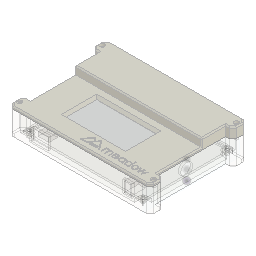
GNSS_Tracker_Enclosure (Autodesk Fusion 360 design; units mm, degrees)
Autodesk Fusion 360 part; units mm, degrees
note: some values were not read from the file. Set by a fixed rule: which sketch regions a step uses.
(part 1 of 2)
sketch "Sketch1" plane through (0, 0, 0) normal (0, 0, 1) x (1, 0, 0) in component "GNSS_PCB"
  line L0 (50, 37.5) -> (-50, 37.5)
  line L1 (-50, 37.5) -> (-50, -37.5)
  line L2 (-50, -37.5) -> (50, -37.5)
  line L3 (50, -37.5) -> (50, 37.5)
  line L4 (50, 37.5) -> (-50, -37.5) construction
  line L5 (-50, 37.5) -> (50, -37.5) construction
  line L6 (0, 37.5) -> (0, -37.5) construction
  line L7 (-50, 0) -> (50, 0) construction
  line L8 (-30.5, 8.425) -> (30.5, 8.425)
  line L9 (30.5, 8.425) -> (30.5, -31.075)
  line L10 (30.5, -31.075) -> (-30.5, -31.075)
  line L11 (-30.5, -31.075) -> (-30.5, 8.425)
  line L12 (-27.5, 1.425) -> (22, 1.425)
  line L13 (22, 1.425) -> (22, -24.075)
  line L14 (22, -24.075) -> (-27.5, -24.075)
  line L15 (-27.5, -24.075) -> (-27.5, 1.425)
  line L16 (-38.5, 35.825) -> (38.5, 35.825)
  line L17 (38.5, 35.825) -> (38.5, 15.175)
  line L18 (38.5, 15.175) -> (-38.5, 15.175)
  line L19 (-38.5, 15.175) -> (-38.5, 35.825)
  line L20 (-33, -37.5) -> (-33, 37.5) construction
  line L21 (40, -37.5) -> (40, 37.5) construction
  line L22 (-28.5, -30.1) -> (-37.5, -30.1)
  line L23 (-37.5, -30.1) -> (-37.5, -37.5)
  line L24 (-37.5, -37.5) -> (-28.5, -37.5)
  line L25 (-28.5, -37.5) -> (-28.5, -30.1)
  line L26 (-28.5, -30.1) -> (-37.5, -37.5) construction
  line L27 (-37.5, -30.1) -> (-28.5, -37.5) construction
  line L28 (42.75, -28.5) -> (37.25, -28.5)
  line L29 (37.25, -28.5) -> (37.25, -40.5)
  line L30 (37.25, -40.5) -> (42.75, -40.5)
  line L31 (42.75, -40.5) -> (42.75, -28.5)
  line L32 (42.75, -28.5) -> (37.25, -40.5) construction
  line L33 (37.25, -28.5) -> (42.75, -40.5) construction
  line L34 (50, -4) -> (-50, -4) construction
  line L35 (-30.5, 3.275) -> (30.5, 3.275)
  line L36 (30.5, 3.275) -> (30.5, -25.925)
  line L37 (30.5, -25.925) -> (-30.5, -25.925)
  line L38 (-30.5, -25.925) -> (-30.5, 3.275)
  point P0 (-47.5, 35)
  point P1 (47.5, 35)
  point P2 (47.5, -35)
  point P3 (-47.5, -35)
  point P4 (-33, -33.8)
  point P5 (40, -34.5)
  dimension "d6" = 75
  dimension "d8" = 100
  dimension "d9" = 2.5
  dimension "d10" = 2.5
  dimension "d19" = 61
  dimension "d20" = 39.5
  dimension "d21" = 30.5
  dimension "d22" = 8.425
  dimension "d23" = 49.5
  dimension "d24" = 25.5
  dimension "d25" = 7
  dimension "d26" = 3
  dimension "d30" = 77
  dimension "d31" = 20.65
  dimension "d32" = 38.5
  dimension "d35" = 35.825
  dimension "d38" = 17
  dimension "d39" = 10
  dimension "d43" = 9
  dimension "d44" = 7.4
  dimension "d45" = 7.4
  dimension "d49" = 5.5
  dimension "d50" = 12
  dimension "d51" = 9
  dimension "d74" = 61
  dimension "d75" = 29.2
  dimension "d76" = 5.15
  constraint horizontal L0
  constraint perpendicular L0 L1
  constraint parallel L0 L2
  constraint parallel L1 L3
  constraint coincident L4 origin
  constraint coincident L5 origin
  constraint midpoint L0 L6.start
  constraint midpoint L2 L6.end
  constraint midpoint L1 L7.start
  constraint midpoint L3 L7.end
  constraint symmetric P0 P1 L6
  constraint symmetric P1 P2 L7
  constraint symmetric P0 P3 L7
  constraint horizontal L8
  constraint vertical L9
  constraint horizontal L10
  constraint vertical L11
  constraint horizontal L12
  constraint vertical L13
  constraint horizontal L14
  constraint vertical L15
  constraint horizontal L16
  constraint vertical L17
  constraint horizontal L18
  constraint vertical L19
  constraint coincident L2 L20.start
  constraint coincident L0 L20.end
  constraint perpendicular L0 L20
  constraint coincident L2 L21.start
  constraint coincident L0 L21.end
  constraint perpendicular L0 L21
  constraint horizontal L22
  constraint perpendicular L22 L23
  constraint parallel L22 L24
  constraint parallel L23 L25
  constraint coincident L26 P4
  constraint coincident L27 P4
  constraint coincident L20 P4
  constraint horizontal L28
  constraint perpendicular L28 L29
  constraint parallel L28 L30
  constraint parallel L29 L31
  constraint coincident L32 P5
  constraint coincident L33 P5
  constraint coincident L21 P5
  constraint coincident L3 L34.start
  constraint coincident L1 L34.end
  constraint perpendicular L1 L34
  constraint horizontal L35
  constraint vertical L36
  constraint horizontal L37
  constraint vertical L38
  constraint coincident L11 L35.start
  measures "d6" distance of L0.end L1.end
  measures "d8" distance of L0.start L0.end
  measures "d9" distance of L0 P0
  measures "d10" distance of L1 P0
  measures "d19" distance of L8.start L8.end
  measures "d20" distance of L8.start L10.end
  measures "d21" distance of L6 L11
  measures "d22" distance of L7 L8
  measures "d23" distance of L12.start L12.end
  measures "d24" distance of L12.start L14.end
  measures "d25" distance of L8 L12
  measures "d26" distance of L11 L15
  measures "d30" distance of L16.start L16.end
  measures "d31" distance of L16.start L18.end
  measures "d32" distance of L6 L19
  measures "d35" distance of L7 L16
  measures "d38" distance of L1 L20
  measures "d39" distance of L3 L21
  measures "d43" distance of L23.end L24.end
  measures "d44" distance of L22.end L23.end
  measures "d45" distance of L2 L22
  measures "d49" distance of L29.end L30.end
  measures "d50" distance of L28.end L29.end
  measures "d51" distance of L2 L28
  measures "d74" distance of L35.start L35.end
  measures "d75" distance of L35.start L37.end
  measures "d76" distance of L8 L35
extrude "Extrude1" add sketch "Sketch1" along normal blind 1.7 contours L0 L1 L2 L3 L8 L9 L10 L11 L22 L23 L25 L28 L29 L31 L36 L38 | L2 L28 L29 L31 | L2 L10 L11 L22 L23 L24 L25 | L9 L10 L11 L22 L25 L37 | L10 L11 L22 L25 | L9 L11 L35 L36 L37 L38 | L8 L9 L11 L35 | L12 L13 L14 L15 | L16 L17 L18 L19 makes body 1 in component "GNSS_PCB"
sketch "Sketch2" plane through (0, 0, 1.7) normal (0, 0, 1) x (-1, 0, 0) in component "GNSS_PCB"
  line L0 (50, 37.5) -> (-50, 37.5)
  line L1 (-50, 37.5) -> (-50, -37.5)
  line L2 (-50, -37.5) -> (50, -37.5)
  line L3 (50, -37.5) -> (50, 37.5)
  line L4 (-37.25, 40.5) -> (-42.75, 40.5)
  line L5 (-37.25, 28.5) -> (-37.25, 40.5)
  line L6 (-42.75, 40.5) -> (-42.75, 28.5)
  line L7 (-40, 37.5) -> (-40, -37.5)
  line L8 (-38.5, -15.175) -> (38.5, -15.175)
  line L9 (-38.5, -35.825) -> (-38.5, -15.175)
  line L10 (38.5, -15.175) -> (38.5, -35.825)
  line L11 (38.5, -35.825) -> (-38.5, -35.825)
  line L12 (-42.75, 28.5) -> (-37.25, 28.5)
  point P0 (47.5, 35)
  point P1 (47.5, -35)
  point P2 (-47.5, -35)
  point P3 (-47.5, 35)
extrude "Extrude2" add sketch "Sketch2" along normal blind 18.5 contours L8 L9 L10 L11 bodies 1 in component "GNSS_PCB"
extrude "Extrude3" add sketch "Sketch2" along normal blind 8.5 contours L0 L5 L7 L12 | L0 L4 L5 L6 | L0 L6 L7 L12 bodies 1 in component "GNSS_PCB"
fillet "Fillet1" radius 10.325 1 edges at (0, 15.175, 20.2) on bodies 1 in component "GNSS_PCB"
fillet "Fillet2" radius 10.325 1 edges at (0, 35.825, 20.2) on bodies 1 in component "GNSS_PCB"
ref_plane "WorkPlane1" through (-5, 0, 3.6) normal (0, 0, 1) x (-1, 0, 0) in component "GNSS_PCB"
sketch "Sketch3" plane through (0, 0, 3.6) normal (0, 0, 1) x (1, 0, 0) in component "GNSS_PCB"
  line L0 (-28.5, -30.1) -> (-37.5, -30.1)
  line L1 (-37.5, -30.1) -> (-37.5, -37.5)
  line L2 (-28.5, -37.5) -> (-28.5, -30.1)
  line L3 (-50, -37.5) -> (50, -37.5)
extrude "Extrude4" add sketch "Sketch3" along normal blind 3.4 separate body makes body 2 in component "GNSS_PCB"
ref_plane "WorkPlane2" through (0, 0, 12.7) normal (0, 0, 1) x (-1, 0, 0) in component "GNSS_PCB"
sketch "Sketch4" plane through (0, 0, 12.7) normal (0, 0, 1) x (1, 0, 0) in component "GNSS_PCB"
  line L0 (-30.5, 8.425) -> (30.5, 8.425)
  line L1 (-30.5, -31.075) -> (-30.5, 8.425)
  line L2 (30.5, 8.425) -> (30.5, -31.075)
  line L3 (30.5, -31.075) -> (-30.5, -31.075)
extrude "Extrude5" add sketch "Sketch4" along normal blind 1.7 separate body makes body 3 in component "GNSS_PCB"
sketch "Sketch5" plane through (0, 0, 14.4) normal (0, 0, 1) x (-1, 0, 0) in component "GNSS_PCB"
  line L0 (-30.5, 31.075) -> (-30.5, -8.425)
  line L1 (-30.5, -8.425) -> (30.5, -8.425)
  line L2 (30.5, -8.425) -> (30.5, 31.075)
  line L3 (30.5, 31.075) -> (-30.5, 31.075)
sketch "Sketch6" plane through (0, 0, 14.4) normal (0, 0, 1) x (-1, 0, 0) in component "GNSS_PCB"
  line L0 (30.5, -3.275) -> (-30.5, -3.275)
  line L1 (-30.5, 25.925) -> (30.5, 25.925)
  line L2 (30.5, 25.925) -> (30.5, -3.275)
  line L3 (-30.5, -3.275) -> (-30.5, 25.925)
extrude "Extrude6" add sketch "Sketch6" along normal blind 1.3 separate body makes body 4 in component "GNSS_PCB"
sketch "Sketch7" plane through (0, 0, 15.7) normal (0, 0, 1) x (-1, 0, 0) in component "GNSS_PCB"
  line L0 (-30.5, -3.275) -> (30.5, -3.275)
  line L1 (30.5, -3.275) -> (30.5, 25.925)
  line L2 (30.5, 25.925) -> (-30.5, 25.925)
  line L3 (-30.5, 25.925) -> (-30.5, -3.275)
  line L4 (-22, 24.075) -> (27.5, 24.075)
  line L5 (-22, -1.425) -> (-22, 24.075)
  line L6 (27.5, 24.075) -> (27.5, -1.425)
  line L7 (27.5, -1.425) -> (-22, -1.425)
hole "Hole1" at (-47.5, -35, 1.7) at (47.5, -35, 1.7) at (-47.5, 35, 1.7) at (47.5, 35, 1.7) direction (0, 0, -1) diameter 2.1 end through all bodies 1 in component "GNSS_PCB"
ref_plane "WorkPlane1" through (0, 0, -3) normal (0, 0, 1) x (1, 0, 0) in component "GNSS_Enclosure_Bottom"
sketch "Sketch1 (2)" plane through (0, 0, -3) normal (0, 0, 1) x (1, 0, 0) in component "GNSS_Enclosure_Bottom"
  line L0 (-50, -37.5) -> (50, -37.5)
  line L1 (50, -37.5) -> (50, 37.5)
  line L2 (50, 37.5) -> (-50, 37.5)
  line L3 (-50, 37.5) -> (-50, -37.5)
  line L4 (51, -38.5) -> (51, 38.5)
  line L5 (51, 38.5) -> (-51, 38.5)
  line L6 (-51, 38.5) -> (-51, -38.5)
  line L7 (-51, -38.5) -> (51, -38.5)
  line L8 (-53, -40.5) -> (53, -40.5)
  line L9 (53, -40.5) -> (53, 40.5)
  line L10 (53, 40.5) -> (-53, 40.5)
  line L11 (-53, 40.5) -> (-53, -40.5)
  circle A0 centre (-47.5, 35) radius 3.5
  circle A1 centre (47.5, 35) radius 3.5
  circle A2 centre (47.5, -35) radius 3.5
  circle A3 centre (-47.5, -35) radius 3.5
  line L12 (-44, 35) -> (-44, 38.5)
  line L13 (-47.5, 31.5) -> (-51, 31.5)
  line L14 (44, 35) -> (44, 38.5)
  line L15 (47.5, 31.5) -> (51, 31.5)
  line L16 (47.5, -31.5) -> (51, -31.5)
  line L17 (44, -35) -> (44, -38.5)
  line L18 (-47.5, -31.5) -> (-51, -31.5)
  line L19 (-44, -35) -> (-44, -38.5)
  point P0 (47.5, 35)
  point P1 (-47.5, 35)
  point P2 (-47.5, -35)
  point P3 (47.5, -35)
  dimension "d87" = 1
  dimension "d88" = 3
  constraint coincident P1 A0.centre
  constraint tangent L5 A0
  constraint coincident P0 A1.centre
  constraint tangent L5 A1
  constraint coincident P3 A2.centre
  constraint tangent L4 A2
  constraint coincident P2 A3.centre
  constraint tangent L7 A3
  constraint coincident A0 L12.start
  constraint coincident L5 L12.end
  constraint tangent A0 L12
  constraint perpendicular L5 L12
  constraint coincident A0 L13.start
  constraint coincident L6 L13.end
  constraint tangent A0 L13
  constraint perpendicular L6 L13
  constraint coincident A1 L14.start
  constraint coincident L5 L14.end
  constraint tangent A1 L14
  constraint perpendicular L5 L14
  constraint coincident A1 L15.start
  constraint coincident L4 L15.end
  constraint tangent A1 L15
  constraint perpendicular L4 L15
  constraint coincident A2 L16.start
  constraint coincident L4 L16.end
  constraint tangent A2 L16
  constraint perpendicular L4 L16
  constraint coincident A2 L17.start
  constraint coincident L7 L17.end
  constraint tangent A2 L17
  constraint perpendicular L7 L17
  constraint coincident A3 L18.start
  constraint coincident L6 L18.end
  constraint tangent A3 L18
  constraint perpendicular L6 L18
  constraint coincident A3 L19.start
  constraint coincident L7 L19.end
  constraint tangent A3 L19
  constraint perpendicular L7 L19
extrude "Extrude1'" add sketch "Sketch1 (2)" against normal blind 2 separate body contours L0 L3 A3 | L0 L3 L6 L7 A3 | L0 L3 A3 | L0 A3 | L3 A3 | L0 A3 L19 | L0 L7 A3 L19 | L3 L6 A3 L18 | L3 A3 L18 | L0 L1 L2 L3 A0 A1 A2 A3 L12 L13 L14 L15 L16 L17 L18 L19 | L0 L7 L17 L19 | L3 L6 L13 L18 | L0 A2 L17 | L0 L7 A2 L17 | L3 L6 A0 L13 | L3 A0 L13 | L0 L1 A2 | L0 A2 | L0 L1 L4 L7 A2 | L3 A0 | L2 L3 A0 | L2 L3 L5 L6 A0 | L0 L1 A2 | L1 A2 L16 | L2 L3 A0 | L2 A0 L12 | L1 A2 | L1 L4 A2 L16 | L1 L4 L15 L16 | L2 A0 | L2 L5 A0 L12 | L2 L5 L12 L14 | L1 A1 L15 | L1 L4 A1 L15 | L2 L5 A1 L14 | L2 A1 L14 | L1 L2 A1 | L1 A1 | L2 A1 | L1 L2 A1 | L1 L2 L4 L5 A1 | L8 L9 L10 L11 makes body 5 in component "GNSS_Enclosure_Bottom"
extrude "Extrude2'" add sketch "Sketch1 (2)" along normal up to surface (18.7 mm away) bodies 5 in component "GNSS_Enclosure_Bottom"
extrude "Extrude3'" add sketch "Sketch1 (2)" along normal blind 3 contours L0 L3 A3 | L0 L3 L6 L7 A3 | L0 L3 A3 | L0 A3 | L3 A3 | L0 A3 L19 | L0 L7 A3 L19 | L3 L6 A3 L18 | L3 A3 L18 | L0 A2 L17 | L0 L7 A2 L17 | L3 L6 A0 L13 | L3 A0 L13 | L0 L1 A2 | L0 A2 | L0 L1 L4 L7 A2 | L3 A0 | L2 L3 A0 | L2 L3 L5 L6 A0 | L1 A2 L16 | L2 A0 L12 | L1 A2 | L1 L4 A2 L16 | L2 A0 | L2 L5 A0 L12 | L1 A1 L15 | L1 L4 A1 L15 | L2 L5 A1 L14 | L2 A1 L14 | L1 L2 A1 | L1 A1 | L2 A1 | L1 L2 L4 L5 A1 picked at (48.0119, -34.834) picked at (-48.3502, 35.8333) picked at (47.0153, 35.6054) bodies 5 in component "GNSS_Enclosure_Bottom"
sketch "Sketch2 (2)" plane through (0, 0, 0) normal (0, 0, 1) x (-1, 0, 0) in component "GNSS_Enclosure_Bottom"
  line L0 (-50, -37.5) -> (-50, -37.4495)
  arc A0 (-50, -37.4495) -> (-49.9495, -37.5) centre (-47.5, -35) ccw
  line L1 (-49.9495, -37.5) -> (-50, -37.5)
  arc A1 (-44, -35) -> (-47.5, -31.5) centre (-47.5, -35) ccw
  line L2 (-47.5, -31.5) -> (-51, -31.5)
  line L3 (-51, -31.5) -> (-51, -38.5)
  line L4 (-51, -38.5) -> (-44, -38.5)
  line L5 (-44, -38.5) -> (-44, -35)
  point P0 (-47.5, 35)
  point P1 (47.5, 35)
  point P2 (47.5, -35)
  point P3 (-47.5, -35)
hole "Hole1'" at (47.5, -35, 0) at (-47.5, -35, 0) at (47.5, 35, 0) at (-47.5, 35, 0) direction (0, 0, -1) diameter 3 depth 3 tip angle 180 bodies 5 in component "GNSS_Enclosure_Bottom"
sketch "Sketch3 (2)" plane through (0, -40.5, 0) normal (0, -1, 0) x (1, 0, 0) in component "GNSS_Enclosure_Bottom"
  line L0 (-53, 15.7) -> (-53, -5)
  line L1 (-53, -5) -> (53, -5)
  line L2 (53, -5) -> (53, 15.7)
  line L3 (53, 15.7) -> (-53, 15.7)
  line L4 (-37.5, 3.6) -> (-28.5, 3.6)
  line L5 (-28.5, 3.6) -> (-28.5, 7)
  line L6 (-28.5, 7) -> (-37.5, 7)
  line L7 (-37.5, 7) -> (-37.5, 3.6)
  line L8 (37.25, 1.7) -> (42.75, 1.7)
  line L9 (42.75, 1.7) -> (42.75, 10.2)
  line L10 (42.75, 10.2) -> (37.25, 10.2)
  line L11 (37.25, 10.2) -> (37.25, 1.7)
  line L12 (36.25, 11.2) -> (36.25, 0.7)
  line L13 (36.25, 0.7) -> (43.75, 0.7)
  line L14 (43.75, 0.7) -> (43.75, 11.2)
  line L15 (43.75, 11.2) -> (36.25, 11.2)
  line L16 (-33, 7) -> (-33, 3.6) construction
  line L17 (-37.5, 5.3) -> (-28.5, 5.3) construction
  line L18 (-26, 10.3) -> (-40, 10.3)
  line L19 (-40, 10.3) -> (-40, 0.3)
  line L20 (-40, 0.3) -> (-26, 0.3)
  line L21 (-26, 0.3) -> (-26, 10.3)
  line L22 (-26, 10.3) -> (-40, 0.3) construction
  line L23 (-40, 10.3) -> (-26, 0.3) construction
  point P0 (-33, 5.3)
  dimension "d102" = 1
  dimension "d107" = 14
  dimension "d108" = 10
  constraint midpoint L6 L16.start
  constraint midpoint L4 L16.end
  constraint midpoint L7 L17.start
  constraint midpoint L5 L17.end
  constraint horizontal L18
  constraint perpendicular L18 L19
  constraint parallel L18 L20
  constraint parallel L19 L21
  constraint coincident L22 P0
  constraint coincident L23 P0
  constraint midpoint L17 P0
  measures "d107" distance of L19.end L20.end
  measures "d108" distance of L18.end L19.end
extrude "Extrude4'" cut sketch "Sketch3 (2)" against normal up to surface (2 mm away) contours L8 L9 L10 L11 | L12 L13 L14 L15 bodies 5 in component "GNSS_Enclosure_Bottom"
extrude "Extrude5'" cut sketch "Sketch3 (2)" against normal up to surface (2 mm away) contours L4 L5 L6 L7 | L18 L19 L20 L21 bodies 5 in component "GNSS_Enclosure_Bottom"
sketch "Sketch1 (3)" plane through (0, 0, 15.7) normal (0, 0, 1) x (-1, 0, 0) in component "GNSS_Enclosure_Top"
  line L0 (-51, -38.5) -> (-51, 38.5)
  line L1 (-51, 38.5) -> (51, 38.5)
  line L2 (51, 38.5) -> (51, -38.5)
  line L3 (51, -38.5) -> (-51, -38.5)
  line L4 (-53, -40.5) -> (53, -40.5)
  line L5 (53, -40.5) -> (53, 40.5)
  line L6 (53, 40.5) -> (-53, 40.5)
  line L7 (-53, 40.5) -> (-53, -40.5)
  line L8 (-38.5, -35.825) -> (-38.5, -15.175)
  line L9 (38.5, -35.825) -> (-38.5, -35.825)
  line L10 (-38.5, -15.175) -> (38.5, -15.175)
  line L11 (38.5, -15.175) -> (38.5, -35.825)
  line L12 (53, -40.5) -> (-53, -40.5)
  line L13 (53, 40.5) -> (53, -40.5)
  line L14 (-53, -40.5) -> (-53, 40.5)
  line L15 (-53, 40.5) -> (53, 40.5)
  line L16 (53, -10.5) -> (-53, -10.5)
  line L17 (-51, 38.5) -> (-51, -38.5)
  line L18 (-51, -38.5) -> (51, -38.5)
  line L19 (51, -38.5) -> (51, 38.5)
  dimension "d111" = 4.675
  dimension "d112" = 4.675
  constraint coincident L13 L16.start
  constraint coincident L14 L16.end
  constraint perpendicular L14 L16
  measures "d111" distance of L4 L9
  measures "d112" distance of L10 L16
extrude "Extrude1''" add sketch "Sketch1 (3)" along normal blind 2 separate body contours L0 L2 L3 L4 L5 L7 L12 L13 L14 L16 L17 L18 L19 | L0 L1 L2 L5 L6 L7 L13 L14 L15 L16 L17 L19 | L0 L1 L2 L16 L17 L19 makes body 6 in component "GNSS_Enclosure_Top"
sketch "Sketch2 (3)" plane through (0, 0, 17.7) normal (0, 0, 1) x (-1, 0, 0) in component "GNSS_Enclosure_Top"
  line L0 (51, -10.5) -> (51, -38.5)
  line L1 (51, -38.5) -> (-51, -38.5)
  line L2 (-51, -38.5) -> (-51, -10.5)
  line L3 (-51, -10.5) -> (51, -10.5)
  line L4 (-53, 40.5) -> (-53, -40.5)
  line L5 (-53, -40.5) -> (53, -40.5)
  line L6 (53, -40.5) -> (53, 40.5)
  line L7 (53, 40.5) -> (-53, 40.5)
  line L8 (-53, -8.5) -> (53, -8.5)
  dimension "d115" = 2
  constraint coincident L4 L8.start
  constraint coincident L6 L8.end
  constraint perpendicular L6 L8
  measures "d115" distance of L3 L8
sketch "Sketch3 (3)" plane through (53, 0, 0) normal (1, 0, 0) x (0, 1, 0) in component "GNSS_Enclosure_Top"
  line L0 (-40.5, 15.7) -> (40.5, 15.7)
  line L1 (40.5, 15.7) -> (40.5, 17.7)
  line L2 (40.5, 17.7) -> (-40.5, 17.7)
  line L3 (-40.5, 17.7) -> (-40.5, 15.7)
  arc A0 (35.825, 9.875) -> (15.175, 9.875) centre (25.5, 9.875) ccw
  line L4 (25.5, 20.2) -> (40.5, 20.2) construction
  line L5 (40.5, 20.2) -> (40.5, 17.7) construction
  line L6 (25.5, 22.2) -> (42.5, 22.2) construction
  line L7 (42.5, 22.2) -> (42.5, 17.7) construction
  constraint midpoint A0 L4.start
  constraint tangent A0 L4
  constraint perpendicular L1 L4
  constraint coincident L1.end L2.start
  constraint perpendicular L2 L5
extrude "Extrude2''" add sketch "Sketch2 (3)" along normal up to surface (4.5 mm away) contours L4 L5 L6 L8 bodies 6 in component "GNSS_Enclosure_Top"
sketch "Sketch4 (2)" plane through (0, 0, 22.2) normal (0, 0, 1) x (-1, 0, 0) in component "GNSS_Enclosure_Top"
  line L0 (51, -38.5) -> (-51, -38.5)
  line L1 (-51, -38.5) -> (-51, -10.5)
  line L2 (-51, -10.5) -> (51, -10.5)
  line L3 (51, -10.5) -> (51, -38.5)
  line L4 (-53, -8.5) -> (-53, -40.5)
  line L5 (-53, -40.5) -> (53, -40.5)
  line L6 (53, -40.5) -> (53, -8.5)
  line L7 (53, -8.5) -> (-53, -8.5)
extrude "Extrude3''" add sketch "Sketch4 (2)" along normal blind 2 contours L0 L1 L2 L3 | L4 L5 L6 L7 bodies 6 in component "GNSS_Enclosure_Top"
sketch "Sketch4 (3)" plane through (53, 0, 0) normal (1, 0, 0) x (0, 1, 0) in component "GNSS_Enclosure_Bottom"
  line L0 (-40.5, 15.7) -> (-40.5, -5)
  line L1 (-40.5, -5) -> (40.5, -5)
  line L2 (40.5, -5) -> (40.5, 15.7)
  line L3 (40.5, 15.7) -> (-40.5, 15.7)
  line L4 (-4, 0) -> (-4, 15.7) construction
  point P0 (-4, 0)
  point P1 (-4, 8.2)
  dimension "d124" = 8.2
  constraint coincident P0 L4.start
  constraint coincident L3 L4.end
  constraint perpendicular L3 L4
  constraint coincident L4 P1
  measures "d124" distance of P0 P1
hole "Hole2" at (53, -4, 8.2) direction (-1, 0, 0) diameter 10 depth 2 tip angle 180 bodies 5 in component "GNSS_Enclosure_Bottom"
sketch "Sketch5 (2)" plane through (0, 0, -5) normal (0, 0, -1) x (1, 0, 0) in component "GNSS_Enclosure_Bottom"
  line L0 (-53, 40.5) -> (-53, -40.5)
  line L1 (-53, -40.5) -> (53, -40.5)
  line L2 (53, -40.5) -> (53, 40.5)
  line L3 (53, 40.5) -> (-53, 40.5)
  line L4 (-53, 40.5) -> (-53, -40.5)
  line L5 (53, -40.5) -> (53, 40.5)
  line L6 (59, -40.5) -> (59, 40.5) construction
  line L7 (-59, 40.5) -> (-59, -40.5) construction
  line L8 (59, -40.5) -> (53, -40.5) construction
  line L9 (59, 40.5) -> (53, 40.5) construction
  line L10 (-59, -40.5) -> (-53, -40.5) construction
  line L11 (-59, 40.5) -> (-53, 40.5) construction
  line L12 (59, -28.5) -> (53, -28.5) construction
  line L13 (56, -40.5) -> (56, -28.5) construction
  line L14 (53, -40.5) -> (59, -40.5)
  line L15 (59, -28.5) -> (59, -40.5)
  line L16 (59, -28.5) -> (53, -28.5)
  line L17 (59, 28.5) -> (53, 28.5)
  line L18 (59, 28.5) -> (59, 40.5)
  line L19 (59, 40.5) -> (53, 40.5)
  line L20 (-59, -28.5) -> (-53, -28.5)
  line L21 (-59, 28.5) -> (-53, 28.5)
  line L22 (-53, -40.5) -> (-59, -40.5)
  line L23 (-59, -28.5) -> (-59, -40.5)
  line L24 (-59, 28.5) -> (-59, 40.5)
  line L25 (-59, 40.5) -> (-53, 40.5)
  line L26 (56, 28.5) -> (56, 40.5) construction
  line L27 (59, 34.5) -> (53, 34.5) construction
  line L28 (-56, -40.5) -> (-56, -28.5) construction
  line L29 (-56, 28.5) -> (-56, 40.5) construction
  point P0 (56, -34.5)
  point P1 (-56, -34.5)
  point P2 (-56, 34.5)
  point P3 (56, 34.5)
  dimension "d129" = 6
  dimension "d130" = 6
  dimension "d131" = 12
  dimension "d132" = 12
  dimension "d133" = 12
  dimension "d134" = 12
  constraint coincident L1.end L2.start
  constraint perpendicular L5 L8
  constraint coincident L2.end L3.start
  constraint perpendicular L5 L9
  constraint coincident L0.end L1.start
  constraint perpendicular L4 L10
  constraint coincident L0.start L3.end
  constraint perpendicular L4 L11
  constraint coincident L6 L12.start
  constraint coincident L2 L12.end
  constraint perpendicular L2 L12
  constraint midpoint L8 L13.start
  constraint midpoint L12 L13.end
  constraint midpoint L13 P0
  constraint coincident L6 L17.start
  constraint coincident L5 L17.end
  constraint perpendicular L5 L17
  constraint coincident L7 L20.start
  constraint coincident L0 L20.end
  constraint perpendicular L0 L20
  constraint coincident L7 L21.start
  constraint coincident L4 L21.end
  constraint perpendicular L4 L21
  constraint midpoint L17 L26.start
  constraint midpoint L9 L26.end
  constraint midpoint L18 L27.start
  constraint coincident L5 L27.end
  constraint perpendicular L5 L27
  constraint midpoint L10 L28.start
  constraint midpoint L20 L28.end
  constraint midpoint L21 L29.start
  constraint midpoint L25 L29.end
  constraint midpoint L28 P1
  constraint midpoint L29 P2
  constraint midpoint L26 P3
  measures "d131" distance of L8 L12
  measures "d132" distance of L9 L17
  measures "d133" distance of L10 L20
  measures "d134" distance of L11 L21
extrude "Extrude6'" add sketch "Sketch5 (2)" against normal up to surface (20.7 mm away) contours L0 L4 L21 L24 L25 | L2 L5 L17 L18 L19 | L0 L4 L20 L22 L23 | L2 L5 L14 L15 L16 bodies 5 in component "GNSS_Enclosure_Bottom"
chamfer "Chamfer1" distance 3 angle 45 8 edges at (59, -40.5, 5.35) (59, 40.5, 5.35) (59, 28.5, 5.35) (59, -28.5, 5.35) (-59, -40.5, 5.35) (-59, -28.5, 5.35) (-59, 28.5, 5.35) (-59, 40.5, 5.35) on bodies 5 in component "GNSS_Enclosure_Bottom"
sketch "Sketch6 (2)" plane through (0, 0, 15.7) normal (0, 0, 1) x (-1, 0, 0) in component "GNSS_Enclosure_Bottom"
  line L0 (-51, -38.5) -> (-51, 38.5)
  line L1 (-51, 38.5) -> (51, 38.5)
  line L2 (51, 38.5) -> (51, -38.5)
  line L3 (51, -38.5) -> (-51, -38.5)
  line L4 (56, -40.5) -> (59, -37.5)
  line L5 (59, -37.5) -> (59, -31.5)
  line L6 (59, -31.5) -> (56, -28.5)
  line L7 (56, -28.5) -> (53, -28.5)
  line L8 (53, -28.5) -> (53, 28.5)
  line L9 (53, 28.5) -> (56, 28.5)
  line L10 (56, 28.5) -> (59, 31.5)
  line L11 (59, 31.5) -> (59, 37.5)
  line L12 (59, 37.5) -> (56, 40.5)
  line L13 (56, 40.5) -> (-56, 40.5)
  line L14 (-56, 40.5) -> (-59, 37.5)
  line L15 (-59, 37.5) -> (-59, 31.5)
  line L16 (-59, 31.5) -> (-56, 28.5)
  line L17 (-56, 28.5) -> (-53, 28.5)
  line L18 (-53, 28.5) -> (-53, -28.5)
  line L19 (-53, -28.5) -> (-56, -28.5)
  line L20 (-56, -28.5) -> (-59, -31.5)
  line L21 (-59, -31.5) -> (-59, -37.5)
  line L22 (-59, -37.5) -> (-56, -40.5)
  line L23 (-56, -40.5) -> (56, -40.5)
  line L24 (-53, -28.5) -> (-53, -40.5)
  line L25 (53, -28.5) -> (53, -40.5)
  point P0 (-56, 34.5)
  point P1 (-56, -34.5)
  point P2 (56, -34.5)
  point P3 (56, 34.5)
  point P4 (-53, -40.5)
  point P5 (53, -40.5)
  constraint coincident L18.end L19.start
  constraint coincident P4 L24.end
  constraint coincident L7.end L8.start
  constraint coincident P5 L25.end
hole "Hole3" at (-56, -34.5, 15.7) at (-56, 34.5, 15.7) at (56, -34.5, 15.7) at (56, 34.5, 15.7) direction (0, 0, -1) diameter 3 depth 3 tip angle 180 bodies 5 in component "GNSS_Enclosure_Bottom"
chamfer "Chamfer2" distance 0.2 distance2 3 8 edges at (-57.3985, 35.0424, 15.7) (54.6015, 35.0424, 15.7) (-48.8985, 35.5424, 0) (-57.3985, -33.9576, 15.7) (54.6015, -33.9576, 15.7) (46.1015, 35.5424, 0) (46.1015, -34.4576, 0) (-48.8985, -34.4576, 0) measured on face at (54.063, -38.254, 15.7) measured on face at (54.063, -38.254, 15.7) measured on face at (-48.9483, 32.2535, 0) measured on face at (54.063, -38.254, 15.7) measured on face at (54.063, -38.254, 15.7) measured on face at (48.9483, 32.2535, 0) measured on face at (48.9483, -32.2535, 0) measured on face at (-50.3319, -34.9626, 0) on bodies 5 in component "GNSS_Enclosure_Bottom"
sketch "Sketch5 (3)" plane through (0, 0, 15.7) normal (0, 0, -1) x (1, 0, 0) in component "GNSS_Enclosure_Top"
  line L0 (-51, -38.5) -> (-51, -10.5)
  line L1 (-51, -10.5) -> (51, -10.5)
  line L2 (51, -10.5) -> (51, -38.5)
  line L3 (51, -38.5) -> (-51, -38.5)
  line L4 (53, -40.5) -> (53, 40.5)
  line L5 (53, 40.5) -> (-53, 40.5)
  line L6 (-53, 40.5) -> (-53, -40.5)
  line L7 (-53, -40.5) -> (53, -40.5)
  circle A0 centre (-56, 34.5) radius 1.7
  circle A1 centre (-56, -34.5) radius 1.7
  line L8 (51, -38.5) -> (51, 38.5)
  line L9 (51, 38.5) -> (-51, 38.5)
  line L10 (-51, 38.5) -> (-51, -38.5)
  line L11 (-51, -38.5) -> (51, -38.5)
  line L12 (-56, -40.5) -> (-59, -37.5)
  line L13 (-59, -37.5) -> (-59, -31.5)
  line L14 (-59, -31.5) -> (-56, -28.5)
  line L15 (-56, -28.5) -> (-53, -28.5)
  line L16 (-53, -28.5) -> (-53, 28.5)
  line L17 (-53, 28.5) -> (-56, 28.5)
  line L18 (-56, 28.5) -> (-59, 31.5)
  line L19 (-59, 31.5) -> (-59, 37.5)
  line L20 (-59, 37.5) -> (-56, 40.5)
  line L21 (-56, 40.5) -> (56, 40.5)
  line L22 (56, 40.5) -> (59, 37.5)
  line L23 (59, 37.5) -> (59, 31.5)
  line L24 (59, 31.5) -> (56, 28.5)
  line L25 (56, 28.5) -> (53, 28.5)
  line L26 (53, 28.5) -> (53, -28.5)
  line L27 (53, -28.5) -> (56, -28.5)
  line L28 (56, -28.5) -> (59, -31.5)
  line L29 (59, -31.5) -> (59, -37.5)
  line L30 (59, -37.5) -> (56, -40.5)
  line L31 (56, -40.5) -> (-56, -40.5)
  circle A2 centre (56, -34.5) radius 1.7
  circle A3 centre (56, 34.5) radius 1.7
extrude "Extrude4''" add sketch "Sketch5 (3)" against normal up to surface (2 mm away) contours L4 L21 L22 L23 L24 L25 | L6 L17 L18 L19 L20 L21 | A0 | A3 bodies 6 in component "GNSS_Enclosure_Top"
extrude "Extrude5''" add sketch "Sketch6 (2)" along normal up to surface (8.5 mm away) contours L4 L5 L6 L7 L23 L25 | L19 L20 L21 L22 L23 L24 bodies 6 in component "GNSS_Enclosure_Top"
sketch "Sketch6 (3)" plane through (0, 0, 15.7) normal (0, 0, 1) x (1, 0, 0) in component "GNSS_Enclosure_Top"
sketch "Sketch7 (2)" plane through (0, 0, 17.7) normal (0, 0, 1) x (-1, 0, 0) in component "GNSS_Enclosure_Top"
  line L0 (-53, -8.5) -> (53, -8.5)
  line L1 (53, -8.5) -> (53, 28.5)
  line L2 (53, 28.5) -> (56, 28.5)
  line L3 (56, 28.5) -> (59, 31.5)
  line L4 (59, 31.5) -> (59, 37.5)
  line L5 (59, 37.5) -> (56, 40.5)
  line L6 (56, 40.5) -> (-56, 40.5)
  line L7 (-56, 40.5) -> (-59, 37.5)
  line L8 (-59, 37.5) -> (-59, 31.5)
  line L9 (-59, 31.5) -> (-56, 28.5)
  line L10 (-56, 28.5) -> (-53, 28.5)
  line L11 (-53, 28.5) -> (-53, -8.5)
  point P0 (56, 34.5)
  point P1 (-56, 34.5)
sketch "Sketch8" plane through (0, 0, 24.2) normal (0, 0, 1) x (-1, 0, 0) in component "GNSS_Enclosure_Top"
  line L0 (53, -8.5) -> (-53, -8.5)
  line L1 (-53, -8.5) -> (-53, -28.5)
  line L2 (-53, -28.5) -> (-56, -28.5)
  line L3 (-56, -28.5) -> (-59, -31.5)
  line L4 (-59, -31.5) -> (-59, -37.5)
  line L5 (-59, -37.5) -> (-56, -40.5)
  line L6 (-56, -40.5) -> (56, -40.5)
  line L7 (56, -40.5) -> (59, -37.5)
  line L8 (59, -37.5) -> (59, -31.5)
  line L9 (59, -31.5) -> (56, -28.5)
  line L10 (56, -28.5) -> (53, -28.5)
  line L11 (53, -28.5) -> (53, -8.5)
  point P0 (56, -34.5)
  point P1 (-56, -34.5)
hole "Hole1''" at (-56, 34.5, 24.2) at (56, 34.5, 24.2) direction (0, 0, -1) diameter 2.3 depth 8.6 tip angle 180 counterbore diameter 4 counterbore depth 2 bodies 6 in component "GNSS_Enclosure_Top"
hole "Hole2'" at (-56, -34.5, 17.7) at (56, -34.5, 17.7) direction (0, 0, -1) diameter 2.3 depth 2 tip angle 180 counterbore diameter 4 counterbore depth 1 bodies 6 in component "GNSS_Enclosure_Top"
sketch "Sketch9" plane through (0, 0, 17.7) normal (0, 0, 1) x (-1, 0, 0) in component "GNSS_Enclosure_Top"
  circle A0 centre (56, 34.5) radius 2
  circle A1 centre (-56, 34.5) radius 2
  line L0 (-53, -8.5) -> (53, -8.5)
  line L1 (53, -8.5) -> (53, 28.5)
  line L2 (53, 28.5) -> (56, 28.5)
  line L3 (56, 28.5) -> (59, 31.5)
  line L4 (59, 31.5) -> (59, 37.5)
  line L5 (59, 37.5) -> (56, 40.5)
  line L6 (56, 40.5) -> (-56, 40.5)
  line L7 (-56, 40.5) -> (-59, 37.5)
  line L8 (-59, 37.5) -> (-59, 31.5)
  line L9 (-59, 31.5) -> (-56, 28.5)
  line L10 (-56, 28.5) -> (-53, 28.5)
  line L11 (-53, 28.5) -> (-53, -8.5)
  line L12 (27.5, -1.425) -> (-22, -1.425)
  line L13 (27.5, 24.075) -> (27.5, -1.425)
  line L14 (-22, 24.075) -> (27.5, 24.075)
  line L15 (-22, -1.425) -> (-22, 24.075)
extrude "Extrude6''" cut sketch "Sketch9" against normal up to surface (2 mm away) contours L12 L13 L14 L15 bodies 6 in component "GNSS_Enclosure_Top"
chamfer "Chamfer1'" distance 2 angle 45 4 edges at (-2.75, 1.425, 17.7) (22, -11.325, 17.7) (-2.75, -24.075, 17.7) (-27.5, -11.325, 17.7) on bodies 6 in component "GNSS_Enclosure_Top"
chamfer "Chamfer2'" distance 1 angle 45 25 edges at (59, -34.5, 17.7) (57.5, -30, 17.7) (54.5, -28.5, 17.7) (53, -10, 17.7) (57.5, -39, 17.7) (0, -40.5, 17.7) (-57.5, -39, 17.7) (-59, -34.5, 17.7) (-57.5, -30, 17.7) (-54.5, -28.5, 17.7) (-53, -10, 17.7) (-53, 8.5, 20.95) (-53, 18.5, 24.2) (0, 8.5, 24.2) (-54.5, 28.5, 24.2) (-57.5, 30, 24.2) (-59, 34.5, 24.2) (-57.5, 39, 24.2) (0, 40.5, 24.2) (57.5, 39, 24.2) (59, 34.5, 24.2) (57.5, 30, 24.2) (54.5, 28.5, 24.2) (53, 18.5, 24.2) (53, 8.5, 20.95) on bodies 6 in component "GNSS_Enclosure_Top"
chamfer "Chamfer3" distance 1 angle 45 20 edges at (0, -40.5, -5) (-57.5, -39, -5) (-59, -34.5, -5) (-57.5, -30, -5) (-54.5, -28.5, -5) (-53, 0, -5) (57.5, -39, -5) (59, -34.5, -5) (57.5, -30, -5) (54.5, -28.5, -5) (53, 0, -5) (54.5, 28.5, -5) (57.5, 30, -5) (59, 34.5, -5) (57.5, 39, -5) (0, 40.5, -5) (-57.5, 39, -5) (-59, 34.5, -5) (-57.5, 30, -5) (-54.5, 28.5, -5) on bodies 5 in component "GNSS_Enclosure_Bottom"
sketch "Sketch10" plane through (0, 0, 17.7) normal (0, 0, 1) x (-1, 0, 0) in component "GNSS_Enclosure_Top"
  line L0 (-24, -3.425) -> (-24, 26.075)
  line L1 (-24, 26.075) -> (29.5, 26.075)
  line L2 (29.5, 26.075) -> (29.5, -3.425)
  line L3 (29.5, -3.425) -> (-24, -3.425)
  line L4 (52, -8.5) -> (52, 29.5)
  line L5 (52, 29.5) -> (55.5858, 29.5)
  line L6 (55.5858, 29.5) -> (58, 31.9142)
  line L7 (58, 31.9142) -> (58, 34.5)
  circle A0 centre (56, 34.5) radius 2
  line L8 (58, 34.5) -> (58, 37.0858)
  line L9 (58, 37.0858) -> (55.5858, 39.5)
  line L10 (55.5858, 39.5) -> (-55.5858, 39.5)
  line L11 (-55.5858, 39.5) -> (-58, 37.0858)
  line L12 (-58, 37.0858) -> (-58, 34.5)
  circle A1 centre (-56, 34.5) radius 2
  line L13 (-58, 34.5) -> (-58, 31.9142)
  line L14 (-58, 31.9142) -> (-55.5858, 29.5)
  line L15 (-55.5858, 29.5) -> (-52, 29.5)
  line L16 (-52, 29.5) -> (-52, -8.5)
  line L17 (-52, -8.5) -> (52, -8.5)
  line L18 (-20.2661, 33.2143) -> (-20.2661, 35.8128)
  line L19 (-20.2661, 35.8128) -> (-19.6706, 35.8128)
  line L20 (-19.6706, 35.8128) -> (-19.6706, 33.2294)
  spline S0 degree 3 poles (-19.6706, 33.2294) (-19.6706, 32.473) (-19.1109, 31.8735) (-18.3752, 31.8735) knots 0 0 0 0 1 1 1 1
  spline S1 degree 3 poles (-18.3752, 31.8735) (-17.6395, 31.8735) (-17.0687, 32.4724) (-17.0687, 33.2294) knots 0 0 0 0 1 1 1 1
  line L21 (-17.0687, 33.2294) -> (-17.0687, 35.8107)
  line L22 (-17.0687, 35.8107) -> (-16.4822, 35.8107)
  line L23 (-16.4822, 35.8107) -> (-16.4822, 33.2294)
  spline S2 degree 3 poles (-16.4822, 33.2294) (-16.4822, 32.473) (-15.9046, 31.8735) (-15.1758, 31.8735) knots 0 0 0 0 1 1 1 1
  spline S3 degree 3 poles (-15.1758, 31.8735) (-14.4469, 31.8735) (-13.8755, 32.473) (-13.8755, 33.2294) knots 0 0 0 0 1 1 1 1
  line L24 (-13.8755, 33.2294) -> (-13.8755, 35.8107)
  line L25 (-13.8755, 35.8107) -> (-13.2979, 35.8107)
  line L26 (-13.2979, 35.8107) -> (-13.2979, 31.4079)
  line L27 (-13.2979, 31.4079) -> (-13.8755, 31.4079)
  line L28 (-13.8755, 31.4079) -> (-13.8755, 32.0605)
  spline S4 degree 3 poles (-13.8755, 32.0605) (-14.2016, 31.6114) (-14.7212, 31.3436) (-15.2762, 31.3385) knots 0 0 0 0 1 1 1 1
  spline S5 degree 3 poles (-15.2762, 31.3385) (-15.9326, 31.3381) (-16.5356, 31.7006) (-16.8432, 32.2805) knots 0 0 0 0 1 1 1 1
  spline S6 degree 3 poles (-16.8432, 32.2805) (-17.1409, 31.7167) (-17.7371, 31.3385) (-18.4715, 31.3385) knots 0 0 0 0 1 1 1 1
  spline S7 degree 3 poles (-18.4715, 31.3385) (-19.4953, 31.3378) (-20.2661, 32.1657) (-20.2661, 33.2143) knots 0 0 0 0 1 1 1 1
  line L29 (-25.0333, 34.1831) -> (-25.5229, 34.3592)
  spline S8 degree 3 poles (-25.5229, 34.3592) (-25.2953, 34.978) (-24.5341, 35.8478) (-23.3521, 35.8396) knots 0 0 0 0 1 1 1 1
  spline S9 degree 3 poles (-23.3521, 35.8396) (-22.3516, 35.8248) (-21.4748, 35.1666) (-21.1813, 34.2099) knots 0 0 0 0 1 1 1 1
  spline S10 degree 3 poles (-21.1813, 34.2099) (-21.121, 34.0032) (-21.0913, 33.7886) (-21.0933, 33.5732) knots 0 0 0 0 1 1 1 1
  spline S11 degree 3 poles (-21.0933, 33.5732) (-21.0779, 32.3729) (-22.0065, 31.3713) (-23.2046, 31.2961) knots 0 0 0 0 1 1 1 1
  spline S12 degree 3 poles (-23.2046, 31.2961) (-24.4027, 31.2209) (-25.4492, 32.0985) (-25.5841, 33.2913) knots 0 0 0 0 1 1 1 1
  spline S13 degree 3 poles (-25.5841, 33.2913) (-25.5912, 33.3289) (-25.5942, 33.3672) (-25.593, 33.4054) knots 0 0 0 0 1 1 1 1
  line L30 (-25.593, 33.4054) -> (-21.7679, 34.1041)
  spline S14 degree 3 poles (-21.7679, 34.1041) (-21.9694, 34.811) (-22.6142, 35.2994) (-23.3493, 35.3019) knots 0 0 0 0 1 1 1 1
  spline S15 degree 3 poles (-23.3493, 35.3019) (-24.1745, 35.3019) (-24.8318, 34.738) (-25.0333, 34.1831) knots 0 0 0 0 1 1 1 1
  spline S16 degree 3 poles (-21.6716, 33.4268) (-21.6716, 33.4797) (-21.6798, 33.5416) (-21.6798, 33.633) knots 0 0 0 0 1 1 1 1
  line L31 (-21.6798, 33.633) -> (-24.9363, 33.0431)
  spline S17 degree 3 poles (-24.9363, 33.0431) (-24.7144, 32.3251) (-24.0506, 31.8356) (-23.2992, 31.8356) knots 0 0 0 0 1 1 1 1
  spline S18 degree 3 poles (-23.2992, 31.8356) (-22.4248, 31.8593) (-21.7158, 32.5518) (-21.6716, 33.4254) knots 0 0 0 0 1 1 1 1
  line L32 (-21.6716, 33.4254) -> (-21.6716, 33.4268)
  line L33 (-30.8656, 31.4079) -> (-30.8656, 35.8128)
  line L34 (-30.8656, 35.8128) -> (-30.288, 35.8128)
  line L35 (-30.288, 35.8128) -> (-30.288, 35.099)
  spline S19 degree 3 poles (-30.288, 35.099) (-29.5994, 35.8815) (-28.4658, 36.0931) (-27.5413, 35.6116) knots 0 0 0 0 1 1 1 1
  spline S20 degree 3 poles (-27.5413, 35.6116) (-26.6169, 35.1302) (-26.1404, 34.08) (-26.3868, 33.0672) knots 0 0 0 0 1 1 1 1
  spline S21 degree 3 poles (-26.3868, 33.0672) (-26.6333, 32.0545) (-27.5391, 31.3407) (-28.5814, 31.3378) knots 0 0 0 0 1 1 1 1
  spline S22 degree 3 poles (-28.5814, 31.3378) (-29.238, 31.3347) (-29.8625, 31.6216) (-30.288, 32.1217) knots 0 0 0 0 1 1 1 1
  line L36 (-30.288, 32.1217) -> (-30.288, 31.4079)
  line L37 (-30.288, 31.4079) -> (-30.8656, 31.4079)
  spline S23 degree 3 poles (-30.2708, 33.6083) (-30.2708, 32.6456) (-29.5351, 31.8893) (-28.5896, 31.8893) knots 0 0 0 0 1 1 1 1
  spline S24 degree 3 poles (-28.5896, 31.8893) (-27.6402, 31.8893) (-26.8706, 32.6589) (-26.8706, 33.6083) knots 0 0 0 0 1 1 1 1
  spline S25 degree 3 poles (-26.8706, 33.6083) (-26.8706, 34.5577) (-27.6402, 35.3273) (-28.5896, 35.3273) knots 0 0 0 0 1 1 1 1
  spline S26 degree 3 poles (-28.5896, 35.3273) (-29.5351, 35.328) (-30.2708, 34.5709) (-30.2708, 33.6104) knots 0 0 0 0 1 1 1 1
  line L38 (-30.2708, 33.6104) -> (-30.2708, 33.6083)
  line L39 (-36.3046, 29.2592) -> (-36.3046, 35.8128)
  line L40 (-36.3046, 35.8128) -> (-35.727, 35.8128)
  line L41 (-35.727, 35.8128) -> (-35.727, 35.099)
  spline S27 degree 3 poles (-35.727, 35.099) (-35.0384, 35.8815) (-33.9048, 36.0931) (-32.9803, 35.6116) knots 0 0 0 0 1 1 1 1
  spline S28 degree 3 poles (-32.9803, 35.6116) (-32.0559, 35.1302) (-31.5794, 34.08) (-31.8258, 33.0672) knots 0 0 0 0 1 1 1 1
  spline S29 degree 3 poles (-31.8258, 33.0672) (-32.0722, 32.0545) (-32.978, 31.3407) (-34.0203, 31.3378) knots 0 0 0 0 1 1 1 1
  spline S30 degree 3 poles (-34.0203, 31.3378) (-34.6769, 31.3347) (-35.3015, 31.6216) (-35.727, 32.1217) knots 0 0 0 0 1 1 1 1
  line L42 (-35.727, 32.1217) -> (-35.727, 29.2592)
  line L43 (-35.727, 29.2592) -> (-36.3046, 29.2592)
  spline S31 degree 3 poles (-35.7098, 33.6104) (-35.7098, 32.6477) (-34.974, 31.8913) (-34.0286, 31.8913) knots 0 0 0 0 1 1 1 1
  spline S32 degree 3 poles (-34.0286, 31.8913) (-33.0831, 31.8913) (-32.3391, 32.6477) (-32.3391, 33.6104) knots 0 0 0 0 1 1 1 1
  spline S33 degree 3 poles (-32.3391, 33.6104) (-32.3391, 34.573) (-33.0831, 35.3294) (-34.0286, 35.3294) knots 0 0 0 0 1 1 1 1
  spline S34 degree 3 poles (-34.0286, 35.3294) (-34.974, 35.3294) (-35.7098, 34.5709) (-35.7098, 33.6104) knots 0 0 0 0 1 1 1 1
  spline S35 degree 3 poles (-37.2445, 33.6104) (-37.2521, 32.3647) (-38.2667, 31.3603) (-39.5124, 31.3653) knots 0 0 0 0 1 1 1 1
  spline S36 degree 3 poles (-39.5124, 31.3653) (-40.7581, 31.3704) (-41.7646, 32.383) (-41.7621, 33.6287) knots 0 0 0 0 1 1 1 1
  spline S37 degree 3 poles (-41.7621, 33.6287) (-41.7595, 34.8744) (-40.749, 35.8829) (-39.5033, 35.8829) knots 0 0 0 0 1 1 1 1
  spline S38 degree 3 poles (-39.5033, 35.8829) (-38.9019, 35.8827) (-38.3254, 35.6428) (-37.9014, 35.2163) knots 0 0 0 0 1 1 1 1
  spline S39 degree 3 poles (-37.9014, 35.2163) (-37.4775, 34.7897) (-37.241, 34.2117) (-37.2445, 33.6104) knots 0 0 0 0 1 1 1 1
  spline S40 degree 3 poles (-41.1928, 33.6104) (-41.1928, 32.6477) (-40.4577, 31.8838) (-39.5122, 31.8838) knots 0 0 0 0 1 1 1 1
  spline S41 degree 3 poles (-39.5122, 31.8838) (-38.5668, 31.8838) (-37.831, 32.6505) (-37.831, 33.6104) knots 0 0 0 0 1 1 1 1
  spline S42 degree 3 poles (-37.831, 33.6104) (-37.831, 34.5703) (-38.575, 35.3294) (-39.5122, 35.3294) knots 0 0 0 0 1 1 1 1
  spline S43 degree 3 poles (-39.5122, 35.3294) (-40.4495, 35.3294) (-41.1928, 34.5709) (-41.1928, 33.6104) knots 0 0 0 0 1 1 1 1
  line L44 (-48.7784, 31.4079) -> (-47.2293, 35.8128)
  line L45 (-47.2293, 35.8128) -> (-46.6469, 35.8128)
  line L46 (-46.6469, 35.8128) -> (-45.4092, 32.1836)
  line L47 (-45.4092, 32.1836) -> (-44.1715, 35.8128)
  line L48 (-44.1715, 35.8128) -> (-43.5939, 35.8128)
  line L49 (-43.5939, 35.8128) -> (-42.0536, 31.4079)
  line L50 (-42.0536, 31.4079) -> (-42.6312, 31.4079)
  line L51 (-42.6312, 31.4079) -> (-43.8834, 34.9938)
  line L52 (-43.8834, 34.9938) -> (-45.1437, 31.4079)
  line L53 (-45.1437, 31.4079) -> (-45.6684, 31.4079)
  line L54 (-45.6684, 31.4079) -> (-46.9295, 34.9938)
  line L55 (-46.9295, 34.9938) -> (-48.1898, 31.4079)
  line L56 (-48.1898, 31.4079) -> (-48.7784, 31.4079)
  line L57 (-1.2957, 35.8073) -> (3.6551, 35.8073)
  spline S44 degree 3 poles (3.6551, 35.8073) (3.767, 35.8073) (3.8693, 35.7438) (3.9191, 35.6436) knots 0 0 0 0 1 1 1 1
  spline S45 degree 3 poles (3.9191, 35.6436) (3.969, 35.5429) (3.9586, 35.4228) (3.8923, 35.3321) knots 0 0 0 0 1 1 1 1
  line L58 (3.8923, 35.3321) -> (-1.1369, 28.5028)
  spline S46 degree 3 poles (-1.1369, 28.5028) (-1.1924, 28.4273) (-1.2804, 28.3826) (-1.3741, 28.3825) knots 0 0 0 0 1 1 1 1
  spline S47 degree 3 poles (-1.3741, 28.3825) (-1.4668, 28.3835) (-1.5537, 28.4281) (-1.6086, 28.5028) knots 0 0 0 0 1 1 1 1
  line L59 (-1.6086, 28.5028) -> (-4.084, 31.8645)
  spline S48 degree 3 poles (-4.084, 31.8645) (-4.1812, 31.9966) (-4.1535, 32.1824) (-4.0221, 32.2805) knots 0 0 0 0 1 1 1 1
  spline S49 degree 3 poles (-4.0221, 32.2805) (-3.9594, 32.3275) (-3.8805, 32.3474) (-3.803, 32.3359) knots 0 0 0 0 1 1 1 1
  spline S50 degree 3 poles (-3.803, 32.3359) (-3.7256, 32.3244) (-3.6559, 32.2824) (-3.6095, 32.2193) knots 0 0 0 0 1 1 1 1
  line L60 (-3.6095, 32.2193) -> (-1.3741, 29.1794)
  line L61 (-1.3741, 29.1794) -> (3.0671, 35.2118)
  line L62 (3.0671, 35.2118) -> (-1.2957, 35.2118)
  spline S51 degree 3 poles (-1.2957, 35.2118) (-1.4602, 35.2118) (-1.5935, 35.3451) (-1.5935, 35.5095) knots 0 0 0 0 1 1 1 1
  spline S52 degree 3 poles (-1.5935, 35.5095) (-1.5935, 35.674) (-1.4602, 35.8073) (-1.2957, 35.8073) knots 0 0 0 0 1 1 1 1
  spline S53 degree 3 poles (-11.3527, 35.8073) (-11.2587, 35.8073) (-11.1704, 35.7626) (-11.1148, 35.6869) knots 0 0 0 0 1 1 1 1
  line L63 (-11.1148, 35.6869) -> (-6.3242, 29.1794)
  line L64 (-6.3242, 29.1794) -> (-1.5336, 35.6869)
  spline S54 degree 3 poles (-1.5336, 35.6869) (-1.4366, 35.8176) (-1.2522, 35.8453) (-1.1211, 35.7488) knots 0 0 0 0 1 1 1 1
  spline S55 degree 3 poles (-1.1211, 35.7488) (-0.9901, 35.65) (-0.9628, 35.4644) (-1.0599, 35.3321) knots 0 0 0 0 1 1 1 1
  line L65 (-1.0599, 35.3321) -> (-6.087, 28.5028)
  spline S56 degree 3 poles (-6.087, 28.5028) (-6.1424, 28.4273) (-6.2305, 28.3827) (-6.3242, 28.3827) knots 0 0 0 0 1 1 1 1
  spline S57 degree 3 poles (-6.3242, 28.3827) (-6.4179, 28.3827) (-6.506, 28.4273) (-6.5614, 28.5028) knots 0 0 0 0 1 1 1 1
  line L66 (-6.5614, 28.5028) -> (-11.5892, 35.3321)
  spline S58 degree 3 poles (-11.5892, 35.3321) (-11.6866, 35.4643) (-11.6593, 35.6502) (-11.528, 35.7488) knots 0 0 0 0 1 1 1 1
  spline S59 degree 3 poles (-11.528, 35.7488) (-11.4774, 35.7867) (-11.4159, 35.8072) (-11.3527, 35.8073) knots 0 0 0 0 1 1 1 1
  spline S60 degree 3 poles (-4.4835, 34.8584) (-4.4585, 34.8301) (-4.4229, 34.8134) (-4.3852, 34.8121) knots 0 0 0 0 1 1 1 1
  spline S61 degree 3 poles (-4.3852, 34.8121) (-4.3475, 34.8108) (-4.311, 34.825) (-4.2841, 34.8515) knots 0 0 0 0 1 1 1 1
  line L67 (-4.2841, 34.8515) -> (-4.2779, 34.8584)
  line L68 (-4.2779, 34.8584) -> (-3.5861, 35.546)
  spline S62 degree 3 poles (-3.5861, 35.546) (-3.5582, 35.5705) (-3.5413, 35.6054) (-3.5395, 35.6426) knots 0 0 0 0 1 1 1 1
  spline S63 degree 3 poles (-3.5395, 35.6426) (-3.5377, 35.6798) (-3.5511, 35.7161) (-3.5765, 35.7433) knots 0 0 0 0 1 1 1 1
  spline S64 degree 3 poles (-3.5765, 35.7433) (-3.5794, 35.7469) (-3.5826, 35.7501) (-3.5861, 35.7529) knots 0 0 0 0 1 1 1 1
  spline S65 degree 3 poles (-3.5861, 35.7529) (-3.6103, 35.7804) (-3.6445, 35.797) (-3.681, 35.7992) knots 0 0 0 0 1 1 1 1
  spline S66 degree 3 poles (-3.681, 35.7992) (-3.7175, 35.8014) (-3.7534, 35.789) (-3.7807, 35.7646) knots 0 0 0 0 1 1 1 1
  line L69 (-3.7807, 35.7646) -> (-3.7917, 35.7529)
  line L70 (-3.7917, 35.7529) -> (-4.3803, 35.1664)
  line L71 (-4.3803, 35.1664) -> (-4.9696, 35.7529)
  spline S67 degree 3 poles (-4.9696, 35.7529) (-4.9964, 35.7807) (-5.0335, 35.7959) (-5.0721, 35.7949) knots 0 0 0 0 1 1 1 1
  spline S68 degree 3 poles (-5.0721, 35.7949) (-5.1105, 35.7944) (-5.1473, 35.7794) (-5.1752, 35.7529) knots 0 0 0 0 1 1 1 1
  spline S69 degree 3 poles (-5.1752, 35.7529) (-5.2317, 35.7008) (-5.236, 35.613) (-5.1848, 35.5556) knots 0 0 0 0 1 1 1 1
  line L72 (-5.1848, 35.5556) -> (-5.1752, 35.546)
  line L73 (-5.1752, 35.546) -> (-4.4835, 34.8584)
  spline S70 degree 3 poles (-4.4835, 34.0972) (-4.4584, 34.069) (-4.4228, 34.0524) (-4.3851, 34.0512) knots 0 0 0 0 1 1 1 1
  spline S71 degree 3 poles (-4.3851, 34.0512) (-4.3474, 34.0501) (-4.3109, 34.0644) (-4.2841, 34.091) knots 0 0 0 0 1 1 1 1
  line L74 (-4.2841, 34.091) -> (-4.2779, 34.0972)
  line L75 (-4.2779, 34.0972) -> (-3.5861, 34.7889)
  spline S72 degree 3 poles (-3.5861, 34.7889) (-3.5582, 34.8135) (-3.5413, 34.8483) (-3.5395, 34.8855) knots 0 0 0 0 1 1 1 1
  spline S73 degree 3 poles (-3.5395, 34.8855) (-3.5377, 34.9227) (-3.5511, 34.9591) (-3.5765, 34.9863) knots 0 0 0 0 1 1 1 1
  spline S74 degree 3 poles (-3.5765, 34.9863) (-3.5795, 34.9896) (-3.5828, 34.9928) (-3.5861, 34.9959) knots 0 0 0 0 1 1 1 1
  spline S75 degree 3 poles (-3.5861, 34.9959) (-3.6104, 35.0232) (-3.6446, 35.0397) (-3.6812, 35.0418) knots 0 0 0 0 1 1 1 1
  spline S76 degree 3 poles (-3.6812, 35.0418) (-3.7177, 35.0439) (-3.7535, 35.0313) (-3.7807, 35.0069) knots 0 0 0 0 1 1 1 1
  spline S77 degree 2 poles (-3.7807, 35.0069) (-3.7883, 35) (-3.7917, 34.9959) knots 0 0 0 1 1 1
  line L76 (-3.7917, 34.9959) -> (-4.3803, 34.4087)
  line L77 (-4.3803, 34.4087) -> (-4.9696, 34.9959)
  spline S78 degree 3 poles (-4.9696, 34.9959) (-4.9965, 35.0233) (-5.0336, 35.0383) (-5.0721, 35.0371) knots 0 0 0 0 1 1 1 1
  spline S79 degree 3 poles (-5.0721, 35.0371) (-5.1105, 35.0374) (-5.1475, 35.0226) (-5.1752, 34.9959) knots 0 0 0 0 1 1 1 1
  spline S80 degree 3 poles (-5.1752, 34.9959) (-5.2313, 34.9436) (-5.2356, 34.8561) (-5.1848, 34.7985) knots 0 0 0 0 1 1 1 1
  line L78 (-5.1848, 34.7985) -> (-5.1752, 34.7889)
  line L79 (-5.1752, 34.7889) -> (-4.4835, 34.0972)
  spline S81 degree 3 poles (-4.4835, 33.3938) (-4.4584, 33.3656) (-4.4228, 33.349) (-4.3851, 33.3478) knots 0 0 0 0 1 1 1 1
  spline S82 degree 3 poles (-4.3851, 33.3478) (-4.3474, 33.3467) (-4.3109, 33.361) (-4.2841, 33.3876) knots 0 0 0 0 1 1 1 1
  line L80 (-4.2841, 33.3876) -> (-4.2779, 33.3938)
  line L81 (-4.2779, 33.3938) -> (-3.5861, 34.0862)
  spline S83 degree 3 poles (-3.5861, 34.0862) (-3.5295, 34.1433) (-3.5295, 34.2354) (-3.5861, 34.2925) knots 0 0 0 0 1 1 1 1
  spline S84 degree 3 poles (-3.5861, 34.2925) (-3.6134, 34.32) (-3.6505, 34.3355) (-3.6893, 34.3355) knots 0 0 0 0 1 1 1 1
  spline S85 degree 3 poles (-3.6893, 34.3355) (-3.728, 34.3355) (-3.7652, 34.32) (-3.7924, 34.2925) knots 0 0 0 0 1 1 1 1
  line L82 (-3.7924, 34.2925) -> (-4.381, 33.7059)
  line L83 (-4.381, 33.7059) -> (-4.9703, 34.2925)
  spline S86 degree 3 poles (-4.9703, 34.2925) (-4.9973, 34.3197) (-5.0344, 34.3344) (-5.0727, 34.333) knots 0 0 0 0 1 1 1 1
  spline S87 degree 3 poles (-5.0727, 34.333) (-5.111, 34.333) (-5.1479, 34.3185) (-5.1759, 34.2925) knots 0 0 0 0 1 1 1 1
  spline S88 degree 3 poles (-5.1759, 34.2925) (-5.2315, 34.24) (-5.2352, 34.1527) (-5.1841, 34.0958) knots 0 0 0 0 1 1 1 1
  line L84 (-5.1841, 34.0958) -> (-5.1745, 34.0862)
  line L85 (-5.1745, 34.0862) -> (-4.4835, 33.3938)
  spline S89 degree 3 poles (-6.428, 34.8584) (-6.4035, 34.8308) (-6.3689, 34.8143) (-6.3321, 34.8124) knots 0 0 0 0 1 1 1 1
  spline S90 degree 3 poles (-6.3321, 34.8124) (-6.2952, 34.8106) (-6.2592, 34.8237) (-6.2321, 34.8487) knots 0 0 0 0 1 1 1 1
  spline S91 degree 3 poles (-6.2321, 34.8487) (-6.2285, 34.8516) (-6.2253, 34.8548) (-6.2224, 34.8584) knots 0 0 0 0 1 1 1 1
  line L86 (-6.2224, 34.8584) -> (-5.5348, 35.546)
  spline S92 degree 3 poles (-5.5348, 35.546) (-5.5068, 35.5705) (-5.49, 35.6054) (-5.4882, 35.6426) knots 0 0 0 0 1 1 1 1
  spline S93 degree 3 poles (-5.4882, 35.6426) (-5.4864, 35.6798) (-5.4997, 35.7161) (-5.5252, 35.7433) knots 0 0 0 0 1 1 1 1
  spline S94 degree 3 poles (-5.5252, 35.7433) (-5.528, 35.7469) (-5.5313, 35.7501) (-5.5348, 35.7529) knots 0 0 0 0 1 1 1 1
  spline S95 degree 3 poles (-5.5348, 35.7529) (-5.5616, 35.7807) (-5.5988, 35.7959) (-5.6373, 35.7949) knots 0 0 0 0 1 1 1 1
  spline S96 degree 3 poles (-5.6373, 35.7949) (-5.6757, 35.7944) (-5.7125, 35.7794) (-5.7404, 35.7529) knots 0 0 0 0 1 1 1 1
  line L87 (-5.7404, 35.7529) -> (-6.3283, 35.1664)
  line L88 (-6.3283, 35.1664) -> (-6.9169, 35.7529)
  spline S97 degree 3 poles (-6.9169, 35.7529) (-6.944, 35.7808) (-6.9812, 35.7966) (-7.0201, 35.7966) knots 0 0 0 0 1 1 1 1
  spline S98 degree 3 poles (-7.0201, 35.7966) (-7.0589, 35.7966) (-7.0961, 35.7808) (-7.1232, 35.7529) knots 0 0 0 0 1 1 1 1
  spline S99 degree 3 poles (-7.1232, 35.7529) (-7.1798, 35.6958) (-7.1798, 35.6038) (-7.1232, 35.5467) knots 0 0 0 0 1 1 1 1
  line L89 (-7.1232, 35.5467) -> (-6.428, 34.8584)
  spline S100 degree 3 poles (-6.428, 34.0972) (-6.4035, 34.0696) (-6.3689, 34.0531) (-6.3321, 34.0513) knots 0 0 0 0 1 1 1 1
  spline S101 degree 3 poles (-6.3321, 34.0513) (-6.2952, 34.0495) (-6.2592, 34.0625) (-6.2321, 34.0875) knots 0 0 0 0 1 1 1 1
  line L90 (-6.2321, 34.0875) -> (-6.2224, 34.0972)
  line L91 (-6.2224, 34.0972) -> (-5.5348, 34.7889)
  spline S102 degree 3 poles (-5.5348, 34.7889) (-5.493, 34.8297) (-5.4805, 34.8919) (-5.5031, 34.9458) knots 0 0 0 0 1 1 1 1
  spline S103 degree 3 poles (-5.5031, 34.9458) (-5.5257, 34.9996) (-5.5789, 35.0342) (-5.6373, 35.033) knots 0 0 0 0 1 1 1 1
  spline S104 degree 3 poles (-5.6373, 35.033) (-5.6757, 35.0333) (-5.7127, 35.0185) (-5.7404, 34.9918) knots 0 0 0 0 1 1 1 1
  line L92 (-5.7404, 34.9918) -> (-6.3283, 34.4045)